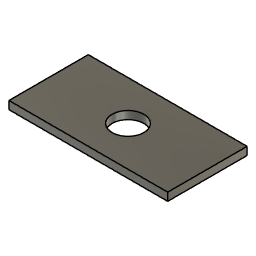
Rectangiular plate with circular hole simultatde (Autodesk Fusion 360 design; units mm, degrees)
Autodesk Fusion 360 part; units mm, degrees
sketch "Sketch1" plane through (0, 0, 0) normal (0, 0, 1) x (1, 0, 0)
  line L0 (-25, 20) -> (75, 20)
  line L1 (75, 20) -> (75, -30)
  line L2 (75, -30) -> (-25, -30)
  line L3 (-25, -30) -> (-25, 20)
  line L4 (-25, 20) -> (75, -30) construction
  line L5 (75, 20) -> (-25, -30) construction
  circle A0 centre (25, -5) radius 10
  dimension "d1" = 100
  dimension "d2" = 50
  dimension "d3" = 20
  constraint horizontal L0
  constraint vertical L1
  constraint horizontal L2
  constraint vertical L3
  constraint midpoint L5 A0.centre
  measures "d1" distance of L0.start L0.end
  measures "d2" distance of L0.end L1.end
  measures "d3" diameter of A0
extrude "Extrude1" add sketch "Sketch1" along normal blind 5
